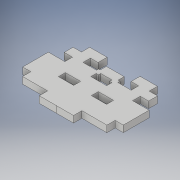
# Autodesk Inventor part: Monster4
Saved by Autodesk Inventor 2019 (Build 230136000, 136)
## iProperties
Created: 2018-12-04
Part Number: Monster4
Material: Generic
Document SubType Name: Modeling
Designer: Administrator
Density: 1 g/cm^3
Appearance: Default
Author: Administrator
Autodesk Inventor part; units mm, degrees
ref_plane "YZ Plane" through (0, 0, 0) normal (1, 0, 0) x (0, 1, 0)
ref_plane "XZ Plane" through (0, 0, 0) normal (0, 1, 0) x (-1, 0, 0)
ref_plane "XY Plane" through (0, 0, 0) normal (0, 0, 1) x (1, 0, 0)
sketch "Sketch1" plane through (0, 0, 0) normal (0, 1, 0) x (-1, 0, 0)
  line L0 (0, 0) -> (419.3723, 0) construction
  line L1 (419.3723, 0) -> (419.3723, -187.719) construction
  line L2 (419.3723, -187.719) -> (0, -187.719) construction
  line L3 (0, -187.719) -> (0, 0) construction
  line L4 (223.6679, -58.3212) -> (216.0306, -58.3212)
  line L5 (216.0306, -58.3212) -> (216.0306, -63.4026)
  line L6 (216.0306, -63.4026) -> (218.2991, -63.4026)
  line L7 (218.2991, -63.4026) -> (218.2991, -65.6711)
  line L8 (218.2991, -65.6711) -> (223.6725, -65.6677)
  line L9 (200.4783, -42.6771) -> (215.133, -42.6771)
  line L10 (215.133, -42.6771) -> (215.133, -49.3831)
  line L11 (215.133, -49.3831) -> (200.4783, -49.3831)
  line L12 (200.4783, -49.3831) -> (200.4783, -42.6771)
  line L13 (207.1541, -17.5006) -> (207.1541, -25.5576)
  line L14 (207.1541, -25.5576) -> (183.0316, -25.5576)
  line L15 (183.0316, -25.5576) -> (183.0316, -33.5176)
  line L16 (183.0316, -33.5176) -> (175.1807, -33.5176)
  line L17 (175.1807, -33.5176) -> (175.1807, -58.3212)
  line L18 (175.1807, -58.3212) -> (191.0462, -58.3212)
  line L19 (191.0462, -58.3212) -> (191.0462, -65.6884)
  line L20 (191.0462, -65.6884) -> (183.0316, -65.6884)
  line L21 (183.0316, -65.6884) -> (183.0316, -74.3282)
  line L22 (183.0316, -74.3282) -> (191.0462, -74.3282)
  line L23 (191.0462, -74.3282) -> (191.0462, -82.3136)
  line L24 (191.0462, -82.3136) -> (207.8056, -82.3136)
  line L25 (207.8056, -82.3136) -> (207.8056, -73.5358)
  line L26 (207.8056, -73.5358) -> (200.4783, -73.5358)
  line L27 (200.4783, -73.5358) -> (200.4783, -66.3936)
  line L28 (200.4783, -66.3936) -> (213.3451, -66.3936)
  line L29 (213.3451, -66.3936) -> (213.3451, -68.5199)
  line L30 (213.3451, -68.5199) -> (215.133, -68.5199)
  line L31 (215.133, -68.5199) -> (215.133, -74.3282)
  line L32 (207.1541, -17.5006) -> (223.642, -17.5006)
  line L33 (223.678, -74.3282) -> (215.133, -74.3282)
  line L34 (223.6679, -58.3212) -> (231.3052, -58.3115)
  line L35 (231.3052, -58.3115) -> (231.3116, -63.3929)
  line L36 (231.3116, -63.3929) -> (229.0431, -63.3958)
  line L37 (229.0431, -63.3958) -> (229.046, -65.6643)
  line L38 (229.046, -65.6643) -> (223.6725, -65.6677)
  line L39 (246.8376, -42.6477) -> (232.1828, -42.6663)
  line L40 (232.1828, -42.6663) -> (232.1913, -49.3723)
  line L41 (232.1913, -49.3723) -> (246.8461, -49.3537)
  line L42 (246.8461, -49.3537) -> (246.8376, -42.6477)
  line L43 (240.1298, -17.4797) -> (240.14, -25.5366)
  line L44 (240.14, -25.5366) -> (264.2625, -25.506)
  line L45 (264.2625, -25.506) -> (264.2726, -33.466)
  line L46 (264.2726, -33.466) -> (272.1235, -33.4561)
  line L47 (272.1235, -33.4561) -> (272.155, -58.2597)
  line L48 (272.155, -58.2597) -> (256.2895, -58.2798)
  line L49 (256.2895, -58.2798) -> (256.2989, -65.647)
  line L50 (256.2989, -65.647) -> (264.3134, -65.6368)
  line L51 (264.3134, -65.6368) -> (264.3244, -74.2766)
  line L52 (264.3244, -74.2766) -> (256.3098, -74.2868)
  line L53 (256.3098, -74.2868) -> (256.32, -82.2722)
  line L54 (256.32, -82.2722) -> (239.5605, -82.2934)
  line L55 (239.5605, -82.2934) -> (239.5494, -73.5156)
  line L56 (239.5494, -73.5156) -> (246.8768, -73.5063)
  line L57 (246.8768, -73.5063) -> (246.8677, -66.3641)
  line L58 (246.8677, -66.3641) -> (234.0008, -66.3805)
  line L59 (234.0008, -66.3805) -> (234.0035, -68.5068)
  line L60 (234.0035, -68.5068) -> (232.2156, -68.509)
  line L61 (232.2156, -68.509) -> (232.223, -74.3174)
  line L62 (240.1298, -17.4797) -> (223.642, -17.5006)
  line L63 (223.678, -74.3282) -> (232.223, -74.3174)
  dimension "d17" = 2.2685
  dimension "d20" = 2.2685
  dimension "d21" = 7.3672
  dimension "d22" = 8.0145
  dimension "d23" = 8.6398
  dimension "d24" = 7.1422
  dimension "d25" = 2.1263
  dimension "d26" = 1.7879
  dimension "d27" = 24.8036
  dimension "d28" = 25.2976
  constraints: 120 end point, 20 perpendicular, 8 point on line, 3 horizontal, 3 parallel, 1 vertical, 2 other
  measures "d17" distance of L5.end L6.end
  measures "d20" distance of L6.end L7.end
  measures "d21" distance of L18.end L19.end
  measures "d22" distance of L19.end L20.end
  measures "d23" distance of L20.end L21.end
  measures "d24" distance of L26.end L27.end
  measures "d25" distance of L28.end L29.end
  measures "d26" distance of L29.end L30.end
  measures "d27" distance of L16.end L17.end
  measures "d28" distance between parallel lines of L17 L12
extrude "Extrusion1" add sketch "Sketch1" along normal blind 6.35
equation "\"d20\" = d17"
body "Solid1"
